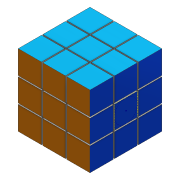
# Autodesk Inventor part: 魔方_状态解释
Saved by Autodesk Inventor 2016 (Build 200138000, 138)
## iProperties
Created: 2019-05-19
Part Number: 魔方_状态解释
Material: 常规
Document SubType Name: Modeling
Designer: oldboy
Density: 1 g/cm^3
Appearance: 默认
Author: oldboy
Autodesk Inventor part; units mm, degrees
ref_plane "YZ Plane" through (0, 0, 0) normal (1, 0, 0) x (0, 1, 0)
ref_plane "XY Plane" through (0, 0, 0) normal (0, 0, 1) x (1, 0, 0)
sketch "草图1" plane through (0, 0, 0) normal (0, 1, 0) x (-1, 0, 0)
  line L0 (-28.5, 28.5) -> (28.5, 28.5)
  line L1 (28.5, 28.5) -> (28.5, -28.5)
  line L2 (28.5, -28.5) -> (-28.5, -28.5)
  line L3 (-28.5, -28.5) -> (-28.5, 28.5)
  line L4 (-28.5, 28.5) -> (28.5, -28.5) construction
  line L5 (28.5, 28.5) -> (-28.5, -28.5) construction
  point P0 (0, 0)
  dimension "d0" = 57
  constraints: 12 end point, 2 midpoint, 2 parallel, 2 perpendicular, 1 horizontal
  measures "d0" distance of L0.end L1.end
extrude "拉伸1" add sketch "草图1" along normal blind 57
sketch "草图2" plane through (-28.5, 0, 28.5) normal (0, 0, 1) x (1, 0, 0)
  line L0 (57, 0) -> (0, 0) projected
  line L1 (57, 0) -> (57, 57) projected
  line L2 (0, 57) -> (57, 57) projected
  line L3 (0, 0) -> (0, 57) projected
  line L4 (0, 57) -> (57, 57) projected
  line L5 (18.5, 57) -> (18.5, 0)
  line L6 (57, 0) -> (0, 0) projected
  line L7 (19.5, 57) -> (19.5, 0)
  line L8 (37.5, 57) -> (37.5, 0)
  line L9 (38.5, 57) -> (38.5, 0)
  point P0 (28.5, 0)
  dimension "d3" = 18.5
  dimension "d4" = 1
  dimension "d5" = 1
  dimension "d6" = 18.5
  constraints: 8 end point, 8 point on line, 3 parallel, 1 vertical
  measures "d3" distance between parallel lines of L5 L3
  measures "d4" distance between parallel lines of L5 L7
  measures "d5" distance between parallel lines of L9 L8
  measures "d6" distance between parallel lines of L1 L9
extrude "拉伸2" cut sketch "草图2" against normal blind 1 contours L0 L8 L2 L9 | L0 L5 L2 L7
mirror "镜像1" about plane through (0, 0, 0) normal (0, 0, 1) of "拉伸2"
sketch "草图3" plane through (0, 57, 0) normal (0, 1, 0) x (1, 0, 0)
  line L0 (-9, 27.5) -> (-10, 27.5) projected
  line L1 (10, 27.5) -> (9, 27.5) projected
  line L2 (-10, -27.5) -> (-9, -27.5) projected
  line L3 (9, -27.5) -> (10, -27.5) projected
  line L4 (-10, 27.5) -> (-10, -27.5)
  line L5 (-9, 27.5) -> (-9, -27.5)
  line L6 (9, 27.5) -> (9, -27.5)
  line L7 (28.5, -28.5) -> (10, -28.5) projected
  line L8 (10, -27.5) -> (9, -27.5) projected
  line L9 (10, -27.5) -> (10, 27.5)
  point P0 (0, 0)
  constraints: 8 end point, 2 parallel, 1 perpendicular, 1 vertical
extrude "拉伸3" cut sketch "草图3" against normal blind 1
ref_plane "工作平面1" through (0, 28.5, 0) normal (0, 1, 0) x (-1, 0, 0)
mirror "镜像2" about plane through (0, 28.5, 0) normal (0, 1, 0) of "拉伸3"
pattern_circular "环形阵列1" count 4 over 360 about axis through (0, -10, 0) along (0, 1, 0) of "拉伸3"
pattern_circular "环形阵列2" count 4 over 360 about axis through (0, -10, 0) along (0, 1, 0) of "拉伸2"
sketch "草图4" plane through (0, 0, 0) normal (0, -1, 0) x (1, 0, 0)
  line L0 (-27.5, -9) -> (-27.5, -10) projected
  line L1 (-27.5, 10) -> (-27.5, 9) projected
  line L2 (27.5, 9) -> (27.5, 10) projected
  line L3 (27.5, -10) -> (27.5, -9) projected
  line L4 (10, -10) -> (27.5, -10) projected
  line L5 (-27.5, -10) -> (27.5, -10)
  line L6 (27.5, -10) -> (27.5, -9)
  line L7 (-27.5, -9) -> (27.5, -9)
  line L8 (-27.5, 9) -> (-10, 9) projected
  line L9 (-27.5, 9) -> (27.5, 9)
  line L10 (-10, 10) -> (-27.5, 10) projected
  line L11 (27.5, 10) -> (-27.5, 10)
  point P0 (0, 0)
  constraints: 10 end point, 2 collinear, 1 horizontal, 1 parallel, 1 perpendicular
extrude "拉伸4" cut sketch "草图4" against normal blind 1
pattern_circular "环形阵列3" count 4 over 360 about axis through (0, -10, 0) along (0, 1, 0) of "拉伸2", "环形阵列2"
sketch "草图5" plane through (28.5, 0, 9) normal (1, 0, 0) x (0, 0, -1)
  line L0 (-19.5, 0) -> (-19.5, 57) projected
  line L1 (-18.5, 56) -> (-18.5, 1) projected
  line L2 (-19.5, 18.5) -> (-18.5, 18.5)
  line L3 (-18.5, 18.5) -> (-18.5, 19.5)
  line L4 (-18.5, 19.5) -> (-19.5, 19.5)
  line L5 (-19.5, 19.5) -> (-19.5, 18.5)
  line L6 (-19.5, 37.5) -> (-18.5, 37.5)
  line L7 (-18.5, 37.5) -> (-18.5, 38.5)
  line L8 (-18.5, 38.5) -> (-19.5, 38.5)
  line L9 (-19.5, 38.5) -> (-19.5, 37.5)
  line L10 (-1, 0) -> (-19.5, 0) projected
  line L11 (-19.5, 57) -> (-1, 57) projected
  point P0 (9, 0)
  dimension "d23" = 1
  dimension "d24" = 18.5
  dimension "d25" = 1
  dimension "d26" = 18.5
  constraints: 16 end point, 4 parallel, 4 point on line, 2 horizontal, 2 perpendicular
  measures "d23" distance between parallel lines of L4 L2
  measures "d24" distance between parallel lines of L10 L2
  measures "d25" distance between parallel lines of L8 L6
  measures "d26" distance between parallel lines of L11 L8
extrude "拉伸5" cut sketch "草图5" against normal blind 60 contours L0 L4 L1 L2 | L0 L8 L1 L6
mirror "镜像3" about plane through (0, 0, 0) normal (0, 0, 1) of "拉伸5"
sketch "草图6" plane through (28.5, 0, 28.5) normal (1, 0, 0) x (0, 0, -1)
  line L0 (1, 38.5) -> (56, 38.5)
  line L1 (56, 38.5) -> (56, 37.5)
  line L2 (56, 37.5) -> (1, 37.5)
  line L3 (1, 37.5) -> (1, 38.5)
  line L4 (1, 18.5) -> (1, 19.5) projected
  line L5 (1, 19.5) -> (56, 19.5)
  line L6 (56, 19.5) -> (56, 18.5)
  line L7 (56, 18.5) -> (1, 18.5)
  line L8 (1, 18.5) -> (1, 19.5)
  point P0 (28.5, 0)
  constraints: 16 end point, 4 parallel, 2 horizontal, 2 perpendicular, 1 point on line
extrude "拉伸6" cut sketch "草图6" against normal blind 1
mirror "镜像4" about plane through (0, 0, 0) normal (1, 0, 0) of "拉伸6"
sketch "草图8" plane through (28.5, 19.5, 9) normal (1, 0, 0) x (0, 0, -1)
  circle A0 centre (9, 9) radius 9 construction
  line L0 (18, 18) -> (0, 18) construction
  line L1 (0, 0) -> (18, 0) construction
  line L2 (0, 18) -> (0, 0) construction
  constraints: 3 tangent, 1 centre point
ref_plane "工作平面2" through (0, 0, 0) normal (0, 0, 1) x (1, 0, 0)
ref_plane "工作平面3" through (0, 0, 0) normal (1, 0, 0) x (0, 1, 0)
